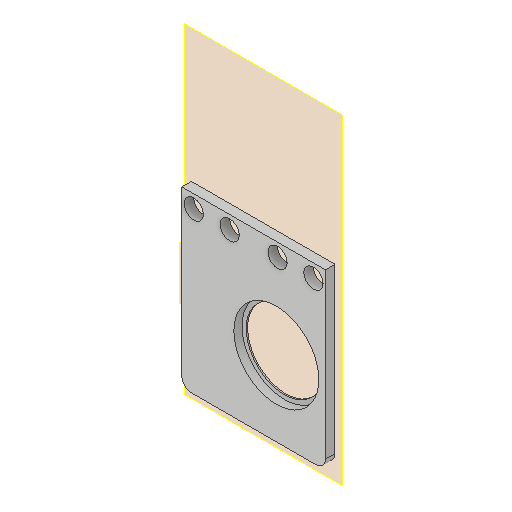
# Autodesk Inventor part: 30_XY_Sample_arm_35mmadapter
Saved by Autodesk Inventor 2022 (Build 260153000, 153)
## iProperties
Created: 2021-06-28
Part Number: 30_XY_Sample_arm_35mmadapter
Material: Generic
Document SubType Name: Modeling
Designer: diederichbenedict
Density: 1 g/cm^3
Appearance: Default
Author: diederichbenedict
Autodesk Inventor part; units mm, degrees
ref_plane "YZ Plane" through (0, 0, 0) normal (1, 0, 0) x (0, 1, 0)
ref_plane "XZ Plane" through (0, 0, 0) normal (0, 1, 0) x (-1, 0, 0)
ref_plane "XY Plane" through (0, 0, 0) normal (0, 0, 1) x (1, 0, 0)
ref_plane "Work Plane1" through (0, 0, 0) normal (0, 0, 1) x (1, 0, 0)
ref_plane "Work Plane2" through (0, 0, 0) normal (0, 0, 1) x (1, 0, 0)
sketch "Sketch2" plane through (0, 0, 0) normal (0, 0, 1) x (1, 0, 0)
  circle A0 centre (24, 55) radius 16 projected
  circle A1 centre (49, 30) radius 4 projected
  circle A2 centre (-1, 80) radius 4 projected
  circle A3 centre (34, 30) radius 4 projected
  circle A4 centre (49, 65) radius 4 projected
  circle A5 centre (14, 80) radius 4 projected
  circle A6 centre (-1, 45) radius 4 projected
  circle A7 centre (-1, 65) radius 4 projected
  circle A8 centre (34, 80) radius 4 projected
  circle A9 centre (49, 45) radius 4 projected
  circle A10 centre (14, 30) radius 4 projected
  circle A11 centre (-1, 30) radius 4 projected
  circle A12 centre (49, 80) radius 4 projected
  arc A13 (54, -29) -> (50, -25) centre (50, -29) ccw projected
  line L0 (50, -25) -> (10, -25) projected
  arc A14 (6, -21) -> (10, -25) centre (10, -21) ccw projected
  line L1 (6, -21) -> (6, 21) projected
  arc A15 (10, 25) -> (6, 21) centre (10, 21) ccw projected
  line L2 (10, 25) -> (52, 25) projected
  line L3 (52, 25) -> (54, 27) projected
  line L4 (54, 27) -> (54, 83) projected
  line L5 (54, 83) -> (52, 85) projected
  line L6 (52, 85) -> (-4, 85) projected
  line L7 (-4, 85) -> (-6, 83) projected
  line L8 (-6, 83) -> (-6, -33) projected
  arc A16 (-6, -33) -> (-2, -37) centre (-2, -33) ccw projected
  line L9 (-2, -37) -> (50, -37) projected
  arc A17 (50, -37) -> (54, -33) centre (50, -33) ccw projected
  line L10 (54, -33) -> (54, -29) projected
  line L11 (54, 35.5093) -> (-6, 35.5093)
  line L12 (54, 27) -> (54, -29)
  circle A18 centre (33.5, 2.5) radius 17.5 construction
  circle A19 centre (33.5, -5.6473) radius 17.75
  point P0 (0, 0)
  dimension "d11" = 35.5
  constraints: 4 end point, 2 point on line, 1 centre point, 1 parallel, 1 perpendicular
  measures "d11" diameter of A19
extrude "Extrusion2" add sketch "Sketch2" along normal blind 4 contours L10 A17 L9 A16 L8 L11 L4 L3 L2 A15 L1 A14 L0 A13 | A13 L0 A14 L1 A15 L2 L3 L12
sketch "Sketch3" plane through (0, 0, 0) normal (0, 0, -1) x (-1, 0, 0)
  circle A0 centre (-33.5, -5.6473) radius 17.75 projected
  circle A1 centre (-33.5, -5.6473) radius 16
  point P0 (0, 0)
  point P1 (-33.5, 2.5)
  dimension "d12" = 32
  constraints: 1 centre point
  measures "d12" diameter of A1
extrude "Extrusion3" add sketch "Sketch3" against normal blind 0.6
body "Solid1"
